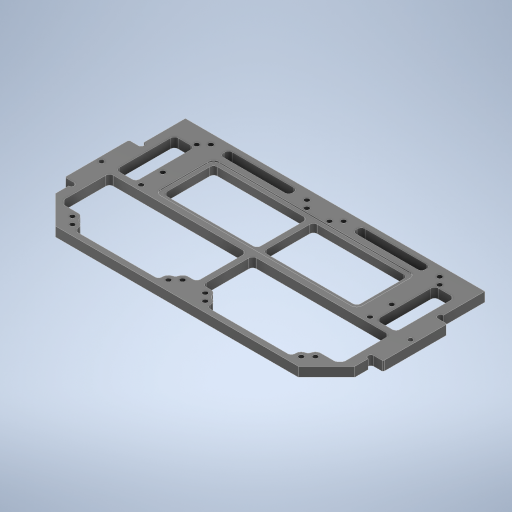
# Autodesk Inventor part: TorsoElectronicBoxBoardMountFrame
Saved by Autodesk Inventor 2024.2 (Build 282272000, 272)
## iProperties
Created: 2024-01-11
Part Number: TorsoElectronicBoxBoardMountFrame
Material: Acetal Resin, Black
Document SubType Name: Modeling
Designer: Masato Kubotera
Density: 1.425 g/cm^3
Appearance: Smooth - Black
Vendor: meviy
Mass: 32.4012 g
Surface Area: 177.402 cm^2
Volume: 22.7377 cm^3
Author: Masato Kubotera
Autodesk Inventor part; units mm, degrees
ref_plane "YZ Plane" through (0, 0, 0) normal (1, 0, 0) x (0, 1, 0)
ref_plane "XZ Plane" through (0, 0, 0) normal (0, 1, 0) x (-1, 0, 0)
ref_plane "XY Plane" through (0, 0, 0) normal (0, 0, 1) x (1, 0, 0)
sketch "Sketch1" plane through (0, 0, 0) normal (0, 0, 1) x (1, 0, 0)
  line L0 (-42, -79.5) -> (42, -79.5)
  line L1 (42, -79.5) -> (42, 79.5)
  line L2 (42, 79.5) -> (-42, 79.5) construction
  line L3 (-42, 79.5) -> (-42, -79.5)
  line L4 (-42, -79.5) -> (42, 79.5) construction
  line L5 (42, -79.5) -> (-42, 79.5) construction
  line L6 (-42, 0) -> (42, 0)
  line L7 (-17, 84.5) -> (17, 84.5)
  line L8 (17, 84.5) -> (17, 79.5)
  line L9 (-17, 84.5) -> (-17, 79.5)
  arc A0 (-20, 79.5) -> (-17, 79.5) centre (-18.5, 79.5) ccw
  line L10 (17, 84.5) -> (17, 79.5)
  arc A1 (17, 79.5) -> (20, 79.5) centre (18.5, 79.5) ccw
  line L11 (0, 79.5) -> (0, 84.5) construction
  line L12 (0, -70) -> (0, 70) construction
  line L13 (-33, 6) -> (33, 6) construction
  line L14 (33, 6) -> (33, 64.5) construction
  line L15 (33, 64.5) -> (-33, 64.5) construction
  line L16 (-33, 64.5) -> (-33, 6) construction
  line L17 (-33, 6) -> (33, 64.5) construction
  line L18 (33, 6) -> (-33, 64.5) construction
  line L19 (-41, 1.75) -> (41, 1.75) construction
  line L20 (41, 1.75) -> (41, 68.75) construction
  line L21 (41, 68.75) -> (-41, 68.75) construction
  line L22 (-41, 68.75) -> (-41, 1.75) construction
  line L23 (-41, 1.75) -> (41, 68.75) construction
  line L24 (41, 1.75) -> (-41, 68.75) construction
  line L25 (-41, 35.25) -> (41, 35.25) construction
  line L26 (5.25, 74.5) -> (26.9289, 74.5)
  arc A2 (36.9, 12.7462) -> (39, 14.7437) centre (37, 14.7437) ccw
  arc A3 (28, 1.5) -> (30, 3.5) centre (28, 3.5) ccw
  line L27 (-42, 79.5) -> (-20, 79.5)
  line L28 (20, 79.5) -> (42, 79.5)
  line L29 (-28, -53.5) -> (-3, -53.5) construction
  line L30 (0, -50.5) -> (0, 50.5) construction
  line L31 (-3, 53.5) -> (-28, 53.5) construction
  line L32 (-31, 50.5) -> (-31, -50.5) construction
  arc A4 (-28, 53.5) -> (-31, 50.5) centre (-28, 50.5) ccw construction
  arc A5 (0, 50.5) -> (-3, 53.5) centre (-3, 50.5) ccw construction
  arc A6 (-31, -50.5) -> (-28, -53.5) centre (-28, -50.5) ccw construction
  arc A7 (-3, -53.5) -> (0, -50.5) centre (-3, -50.5) ccw construction
  line L33 (-31, 0) -> (0, 0) construction
  circle A8 centre (-33, 6) radius 3 construction
  line L34 (-15.5, 53.5) -> (-15.5, -53.5) construction
  line L35 (5.25, 1.5) -> (28, 1.5)
  arc A9 (5.25, 74.5) -> (3.25, 72.5) centre (5.25, 72.5) ccw
  line L36 (-27, 1.5) -> (-4, 1.5)
  line L37 (-2, 3.5) -> (-2, 49.5)
  line L38 (-4, 51.5) -> (-27, 51.5)
  line L39 (-29, 49.5) -> (-29, 3.5)
  arc A10 (-29, 3.5) -> (-27, 1.5) centre (-27, 3.5) ccw
  arc A11 (-4, 1.5) -> (-2, 3.5) centre (-4, 3.5) ccw
  arc A12 (-2, 49.5) -> (-4, 51.5) centre (-4, 49.5) ccw
  arc A13 (-27, 51.5) -> (-29, 49.5) centre (-27, 49.5) ccw
  arc A14 (33.8266, 60.0766) -> (36.9, 57.7538) centre (36.75, 60.75) ccw
  arc A15 (39, 55.7563) -> (36.9, 57.7538) centre (37, 55.7563) ccw
  line L40 (39, 55.7563) -> (39, 14.7437)
  arc A16 (36.9, 12.7462) -> (33.8266, 10.4234) centre (36.75, 9.75) ccw
  line L41 (-31.1, 0) -> (-31.1, 50.6)
  line L42 (-28.1, 53.6) -> (-2.9, 53.6)
  line L43 (0.1, 50.6) -> (0.1, 0)
  arc A17 (0.1, 50.6) -> (-2.9, 53.6) centre (-2.9, 50.6) ccw
  arc A18 (-28.1, 53.6) -> (-31.1, 50.6) centre (-28.1, 50.6) ccw
  arc A19 (3.25, 3.5) -> (5.25, 1.5) centre (5.25, 3.5) ccw
  line L44 (-29.1, 63.75) -> (-1.9, 63.75)
  line L45 (0.1, 65.75) -> (0.1, 72.5)
  line L46 (-1.9, 74.5) -> (-29.1, 74.5)
  line L47 (-31.1, 72.5) -> (-31.1, 65.75)
  line L48 (-37, 16.9) -> (-36.25, 16.9)
  line L49 (-34.25, 18.9) -> (-34.25, 51.6)
  line L50 (-36.25, 53.6) -> (-37, 53.6)
  line L51 (-39, 51.6) -> (-39, 18.9)
  circle A20 centre (-36.75, 9.75) radius 3 construction
  circle A21 centre (-36.75, 60.75) radius 3 construction
  arc A22 (-31.1, 65.75) -> (-29.1, 63.75) centre (-29.1, 65.75) ccw
  arc A23 (-1.9, 63.75) -> (0.1, 65.75) centre (-1.9, 65.75) ccw
  arc A24 (0.1, 72.5) -> (-1.9, 74.5) centre (-1.9, 72.5) ccw
  arc A25 (-29.1, 74.5) -> (-31.1, 72.5) centre (-29.1, 72.5) ccw
  arc A26 (-34.25, 51.6) -> (-36.25, 53.6) centre (-36.25, 51.6) ccw
  arc A27 (-37, 53.6) -> (-39, 51.6) centre (-37, 51.6) ccw
  arc A28 (-39, 18.9) -> (-37, 16.9) centre (-37, 18.9) ccw
  arc A29 (-36.25, 16.9) -> (-34.25, 18.9) centre (-36.25, 18.9) ccw
  line L52 (27, 79.5) -> (42, 64.5)
  line L53 (29.4142, 72.8431) -> (28.3431, 73.9142)
  arc A30 (30, 71.4289) -> (29.4142, 72.8431) centre (28, 71.4289) ccw
  arc A31 (28.3431, 73.9142) -> (26.9289, 74.5) centre (26.9289, 72.5) ccw
  circle A32 centre (33, 6) radius 3 construction
  line L54 (0.25, 9.75) -> (36.75, 9.75) construction
  line L55 (36.75, 9.75) -> (36.75, 60.75) construction
  line L56 (36.75, 60.75) -> (0.25, 60.75) construction
  line L57 (0.25, 60.75) -> (0.25, 9.75) construction
  line L58 (0.25, 9.75) -> (36.75, 60.75) construction
  line L59 (36.75, 9.75) -> (0.25, 60.75) construction
  arc A33 (32.3266, 8.9234) -> (30, 6) centre (33, 6) ccw
  line L60 (30, 3.5) -> (30, 6)
  arc A34 (33.8828, 61.6328) -> (36.9, 57.7538) centre (36.75, 60.75) ccw
  arc A35 (30, 64.5) -> (32.3266, 61.5766) centre (33, 64.5) ccw
  line L61 (30, 71.4289) -> (30, 64.5)
  line L62 (3.25, 3.5) -> (3.25, 72.5)
  circle A36 centre (0.25, 60.75) radius 3 construction
  arc A37 (33.8266, 60.0766) -> (32.3266, 61.5766) centre (31.8776, 59.6276) ccw
  arc A38 (32.3266, 8.9234) -> (33.8266, 10.4234) centre (31.8776, 10.8724) ccw
  point P0 (0, 0)
  point P1 (0, 35.25)
  point P2 (0, 82)
  point P3 (-31, -53.5)
  point P4 (0, -53.5)
  point P5 (-31.1, 63.75)
  point P6 (0.1, 74.5)
  point P7 (0.1, 63.75)
  point P8 (-31.1, 74.5)
  point P9 (-39, 16.9)
  point P10 (-34.25, 53.6)
  point P11 (-34.25, 16.9)
  point P12 (-39, 53.6)
  point P13 (18.5, 35.25)
  point P14 (-11.25, 60.75)
  dimension "d1" = 159
  dimension "d2" = 1.5
  dimension "d3" = 5
  dimension "d36" = 25
  dimension "d42" = 58.5
  dimension "d43" = 66
  dimension "d44" = 82
  dimension "d45" = 67
  dimension "d67" = 5
  dimension "d70" = 42
  dimension "d71" = 84
  dimension "d73" = 25
  dimension "d75" = 12
  dimension "d95" = 3
  dimension "d97" = 31
  dimension "d100" = 107
  dimension "d102" = 6
  dimension "d108" = 3
  dimension "d114" = 2
  dimension "d115" = 2
  dimension "d116" = 3
  dimension "d118" = 6
  dimension "d122" = 2
  dimension "d123" = 0.1
  dimension "d124" = 0.1
  dimension "d147" = 15
  dimension "d148" = 45
  dimension "d150" = 3
  dimension "d151" = 51
  dimension "d153" = 36.5
  dimension "d156" = 25.5
  dimension "d158" = 2
  dimension "d159" = 11.5
  dimension "d160" = 19.5
  constraints: 126 end point, 70 point on circle, 55 tangent, 39 centre point, 31 point on line, 30 equal radius, 20 midpoint, 15 parallel, 13 coincident, 13 horizontal, 10 vertical, 9 symmetric about line, 8 collinear, 7 perpendicular, 10 other
  measures "d1" distance of L1.end L0.end
  measures "d2" radius of A0
  measures "d3" distance of L7.start L9.end
  measures "d36" distance between parallel lines of L8 L1
  measures "d42" distance of L15.end L13.start
  measures "d43" distance of L14.end L15.end
  measures "d44" distance of L21.end L20.end
  measures "d45" distance of L19.end L20.end
  measures "d67" distance between parallel lines of L2 L26
  measures "d70" distance between parallel lines of L1 L12
  measures "d71" distance between parallel lines of L1 L3
  measures "d73" distance between parallel lines of L9 L3
  measures "d75" diameter of point (-33, 6) L6
  measures "d95" radius of A4
  measures "d97" distance of point (-31, -53.5) point (0, -53.5)
  measures "d100" distance between parallel lines of L31 L29
  measures "d102" diameter of A8
  measures "d108" diameter of L35 L6
  measures "d114" distance between parallel lines of L30 L37
  measures "d115" distance between parallel lines of L31 L38
  measures "d116" distance between parallel lines of L1 L40
  measures "d118" diameter of A16
  measures "d122" radius of A3
  measures "d123" distance between parallel lines of L43 L30
  measures "d124" distance between parallel lines of L42 L31
  measures "d147" distance of L1.end L52.end
  measures "d148" angle of L1 L52
  measures "d150" distance between parallel lines of L52 L53
  measures "d151" distance of A14.centre point (36.75, 9.75)
  measures "d153" distance of L55.end L56.end
  measures "d156" distance of point (-11.25, 60.75) A21.centre
  measures "d158" distance from line of L32 point (-33, 6)
  measures "d159" distance of point (0.25, 60.75) point (-11.25, 60.75)
  measures "d160" diameter of point (36.75, 9.75) L6
extrude "Extrusion1" add sketch "Sketch1" against normal blind 5 contours L3 L27 A0 L9 L7 L8 A1 L28 L52 L1 L6 L43 A17 L42 A18 L41 | L41 A18 L42 A17 L43 L6
extrude "Extrusion2" cut sketch "Sketch1" against normal blind 0.7 contours L41 A18 L42 A17 L43 L6
chamfer "C0.5" distance 0.5 angle 45 2 edges at (17, 84.5, -2.5) (-17, 84.5, -2.5)
hole "M3" at (-33, 6, 0) at (-33, 64.5, 0) at (33, 6, 0) at (33, 64.5, 0) at (36.75, 9.75, 0) at (36.75, 60.75, 0) at (-36.75, 9.75, 0) at (-36.75, 60.75, 0) at (0.25, 60.75, 0) at (-11.25, 60.75, 0) direction (0, 0, -1) diameter 2.459 end through all thread size "M3x0.5" class "6H" standard "ANSI Metric M Profile"
hole "Phi2.5" at (0, 82, 0) direction (0, 0, -1) diameter 2.5 end through all
mirror "Mirror1" about plane through (0, 0, 0) normal (0, 1, 0)
ref_plane "Work Plane1" through (-15.5, 53.5, 0) normal (-1, 0, 0) x (0, 0, 1)
body "Solid1"
